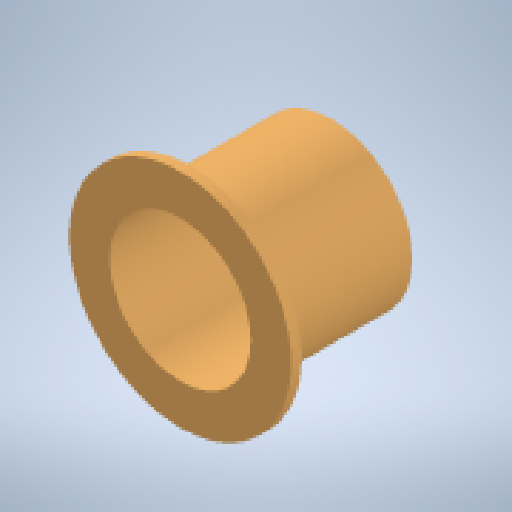
# Autodesk Inventor part: Coussinets
Saved by Autodesk Inventor 2023.2 (Build 272271030, 271C)
## iProperties
Created: 2023-03-16
Part Number: Coussinets
Material: Stainless Steel
Document SubType Name: Modeling
Designer: thuil
Density: 8 g/cm^3
Appearance: Semi-Polished
Author: thuil
Autodesk Inventor part; units mm, degrees
ref_plane "YZ Plane" through (0, 0, 0) normal (1, 0, 0) x (0, 1, 0)
ref_plane "XZ Plane" through (0, 0, 0) normal (0, 1, 0) x (-1, 0, 0)
ref_plane "XY Plane" through (0, 0, 0) normal (0, 0, 1) x (1, 0, 0)
sketch "Esquisse1" plane through (0, 0, 0) normal (0, 0, 1) x (1, 0, 0)
  circle A0 centre (0, 0) radius 7
  circle A1 centre (0, 0) radius 8
  dimension "d0" = 14
  dimension "d1" = 16
  constraints: 2 centre point, 2 coincident
  measures "d0" diameter of A0
  measures "d1" diameter of A1
extrude "Extrusion1" add sketch "Esquisse1" along normal blind 14
sketch "Esquisse2" plane through (0, 0, 14) normal (0, 0, 1) x (1, 0, 0)
  circle A0 centre (0, 0) radius 11
  circle A1 centre (0, 0) radius 7
  dimension "d4" = 22
  constraints: 2 centre point, 2 coincident
  measures "d4" diameter of A0
extrude "Extrusion2" add sketch "Esquisse2" along normal blind 1
sketch "Sketch5" plane through (0, 0, 0) normal (0, 0, -1) x (-1, 0, 0)
  point P0 (0, 0)
